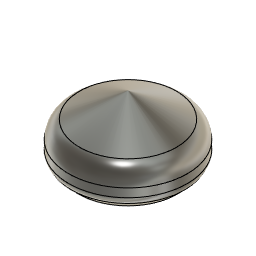
ORS (Autodesk Fusion 360 archive; units mm, degrees)
design "ORS_Button_Pin"
Autodesk Fusion 360 part; units mm, degrees
sketch "Main Body Sketch" plane through (0, 0, 0) normal (0, 0, 1) x (1, 0, 0)
  circle A0 centre (0, 0) radius 3
  dimension "d1" = 6
  constraint coincident A0.centre origin
  measures "d1" diameter of A0
extrude "Extrude1" add sketch "Main Body Sketch" along normal blind 1.75
sketch "Pin Point Sketch" plane through (0, 0, 0) normal (0, 1, 0) x (1, 0, 0)
  line L0 (-3, -1.75) -> (3, -1.75)
  line L1 (3, -1.75) -> (0, -3.29)
  line L2 (0, -3.29) -> (0, -1.75)
  dimension "d4" = 1.54
  constraint coincident L0.end L1.start
  constraint midpoint L0 L2.end
  constraint perpendicular L0 L2
  measures "d4" distance of L1.end L2.end
revolve "Revolve1" add sketch "Pin Point Sketch" angle 360 about axis through (0, 0, 0) along (0, 0, -1)
fillet "Fillet1" radius 1 1 edges at (-2.797, -1.0848, 1.75)
chamfer "Chamfer1" distance 0.5 angle 45 1 edges at (-2.797, -1.0848, 0)
fillet "Fillet2" radius 0.5 1 edges at (-2.797, 1.0848, 0.5)
named bodies: "ORS_Button_Pin"

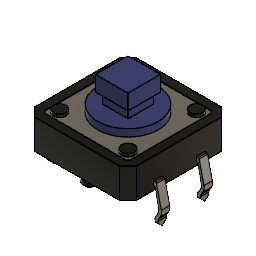
design "OMRON_B3F_5050 v3"
Autodesk Fusion 360 part; units mm, degrees
sketch "Sketch2" plane through (0, 0, 0) normal (0, 0, 1) x (1, 0, 0)
  line L0 (6, 6) -> (-6, 6)
  line L1 (-6, 6) -> (-6, -6)
  line L2 (-6, -6) -> (6, -6)
  line L3 (6, -6) -> (6, 6)
  line L4 (6, 6) -> (-6, -6) construction
  line L5 (-6, 6) -> (6, -6) construction
  circle A0 centre (0.0239, -4.5) radius 0.8
  circle A1 centre (0.0239, 4.5) radius 0.8
  line L6 (-6, 0) -> (6, 0) construction
  line L7 (0, 6) -> (0, -6) construction
  circle A2 centre (0, 0) radius 3.55
  line L8 (1.9, 1.9) -> (-1.9, 1.9)
  line L9 (-1.9, 1.9) -> (-1.9, -1.9)
  line L10 (-1.9, -1.9) -> (1.9, -1.9)
  line L11 (1.9, -1.9) -> (1.9, 1.9)
  line L12 (1.9, 1.9) -> (-1.9, -1.9) construction
  line L13 (-1.9, 1.9) -> (1.9, -1.9) construction
  line L14 (5, 6) -> (6, 5)
  line L15 (-6, 5) -> (-5, 6)
  line L16 (-6, -5) -> (-5, -6)
  line L17 (6, -5) -> (5, -6)
  line L18 (-5, 5) -> (5, 5)
  line L19 (5, 5) -> (5, -5)
  line L20 (5, -5) -> (-5, -5)
  line L21 (-5, -5) -> (-5, 5)
  line L22 (-5, 5) -> (5, -5) construction
  line L23 (5, 5) -> (-5, -5) construction
  line L24 (-4, 4) -> (4, 4) construction
  line L25 (4, 4) -> (4, -4) construction
  line L26 (4, -4) -> (-4, -4) construction
  line L27 (-4, -4) -> (-4, 4) construction
  line L28 (-4, 4) -> (4, -4) construction
  line L29 (4, 4) -> (-4, -4) construction
  circle A3 centre (-4, 4) radius 0.75
  circle A4 centre (4, 4) radius 0.75
  circle A5 centre (4, -4) radius 0.75
  circle A6 centre (-4, -4) radius 0.75
  line L30 (-4.75, -5) -> (-5, -4.75)
  line L31 (-4.75, 5) -> (-5, 4.75)
  line L32 (4.75, 5) -> (5, 4.75)
  line L33 (5, -4.75) -> (4.75, -5)
  line L34 (-6, -2.5) -> (6, -2.5) construction
  line L35 (-6, 2.5) -> (6, 2.5) construction
  line L36 (-1.5, -1.5) -> (1.5, -1.5)
  line L37 (1.5, -1.5) -> (1.5, 1.5)
  line L38 (1.5, 1.5) -> (-1.5, 1.5)
  line L39 (-1.5, 1.5) -> (-1.5, -1.5)
  line L40 (-1.5, -1.5) -> (1.5, 1.5) construction
  line L41 (1.5, -1.5) -> (-1.5, 1.5) construction
  dimension "d3" = 12
  dimension "d4" = 12
  dimension "d5" = 9
  dimension "d6" = 1.6
  dimension "d7" = 7.1
  dimension "d12" = 3.8
  dimension "d13" = 3.8
  dimension "d16" = 1
  dimension "d17" = 1
  dimension "d18" = 1
  dimension "d19" = 1
  dimension "d20" = 10
  dimension "d21" = 10
  dimension "d22" = 8
  dimension "d23" = 8
  dimension "d24" = 1.5
  dimension "d30" = 0.25
  dimension "d31" = 0.25
  dimension "d32" = 0.25
  dimension "d33" = 0.25
  dimension "d37" = 5
  dimension "d46" = 3
  dimension "d47" = 3
  constraint perpendicular L0 L1
  constraint parallel L0 L2
  constraint parallel L1 L3
  constraint horizontal L0
  constraint coincident L4 A2.centre
  constraint coincident L5 A2.centre
  constraint coincident A2.centre origin
  constraint midpoint L1 L6.start
  constraint midpoint L3 L6.end
  constraint midpoint L0 L7.start
  constraint midpoint L2 L7.end
  constraint equal A0 A1
  constraint symmetric A0 A1 L6
  constraint perpendicular L8 L9
  constraint parallel L8 L10
  constraint parallel L9 L11
  constraint horizontal L8
  constraint coincident L12 A2.centre
  constraint coincident L13 A2.centre
  constraint coincident L0 L14.start
  constraint coincident L3 L14.end
  constraint perpendicular L4 L14
  constraint coincident L1 L15.start
  constraint coincident L0 L15.end
  constraint perpendicular L5 L15
  constraint coincident L1 L16.start
  constraint coincident L2 L16.end
  constraint perpendicular L4 L16
  constraint coincident L3 L17.start
  constraint coincident L2 L17.end
  constraint perpendicular L5 L17
  constraint perpendicular L18 L19
  constraint parallel L18 L20
  constraint parallel L19 L21
  constraint horizontal L18
  constraint coincident L22 A2.centre
  constraint coincident L23 A2.centre
  constraint perpendicular L24 L25
  constraint parallel L24 L26
  constraint parallel L25 L27
  constraint horizontal L24
  constraint coincident L28 A2.centre
  constraint coincident L29 A2.centre
  constraint coincident L24.start L27.end
  constraint coincident L24.end L25.start
  constraint coincident L25.end L26.start
  constraint coincident L26.end L27.start
  constraint equal A4 A5
  constraint equal A3 A4
  constraint equal A3 A6
  constraint coincident L20 L30.start
  constraint coincident L21 L30.end
  constraint perpendicular L4 L30
  constraint coincident L18 L31.start
  constraint coincident L21 L31.end
  constraint perpendicular L5 L31
  constraint coincident L18 L32.start
  constraint coincident L19 L32.end
  constraint perpendicular L23 L32
  constraint coincident L19 L33.start
  constraint coincident L20 L33.end
  constraint perpendicular L22 L33
  constraint coincident L1 L34.start
  constraint coincident L3 L34.end
  constraint perpendicular L3 L34
  constraint coincident L1 L35.start
  constraint coincident L3 L35.end
  constraint perpendicular L3 L35
  constraint symmetric L6 L34 L35
  constraint perpendicular L36 L37
  constraint parallel L36 L38
  constraint parallel L37 L39
  constraint horizontal L36
  constraint coincident L40 A2.centre
  constraint coincident L41 A2.centre
  measures "d3" distance of L1.end L2.end
  measures "d4" distance of L0.end L1.end
  measures "d5" distance of A0.centre A1.centre
  measures "d6" diameter of A0
  measures "d7" diameter of A2
  measures "d12" distance of L9.end L10.end
  measures "d13" distance of L8.end L9.end
  measures "d16" distance of L3 L14.start
  measures "d17" distance of L2 L17.start
  measures "d18" distance of L1 L16.end
  measures "d19" distance of L1 L15.end
  measures "d20" distance of L19.end L20.end
  measures "d21" distance of L18.end L19.end
  measures "d22" distance of L25.end L26.end
  measures "d23" distance of L24.end L25.end
  measures "d24" diameter of A4
  measures "d30" distance of L21 L30.start
  measures "d31" distance of L21 L31.start
  measures "d32" distance of L19 L32.start
  measures "d33" distance of L19 L33.end
  measures "d37" distance of L34 L35
  measures "d46" distance of L37.end L38.end
  measures "d47" distance of L36.end L37.end
extrude "Extrude1" add sketch "Sketch2" along normal blind 3.5 contours L0 L1 L2 L3 L14 L15 L16 L17 | A0 L20 | A0 A1 L18 L19 L20 L21 L30 L31 L32 L33 | A0 L20 | L20 L21 L30 | L19 L20 L33 | L18 L21 L31 | L18 L19 L32 | A1 L18 | A1 L18 | A2 | L8 L9 L10 L11 | A3 | A4 | A5 | A6 | L36 L37 L38 L39
sketch "Sketch3" plane through (0, 0, 0) normal (0, 1, 0) x (1, 0, 0)
  line L0 (0, 0) -> (0.0239, -6.3307) construction
  constraint coincident L0.start origin
ref_plane "WorkPlane1" through (0, 2.5, 0) normal (0, -1, 0) x (1, 0, 0)
extrude "Extrude2" add sketch "Sketch2" along normal blind 4.3 contours A2 | L8 L9 L10 L11 | L36 L37 L38 L39
extrude "Extrude3" add sketch "Sketch2" along normal blind 7.3 contours L36 L37 L38 L39
extrude "Extrude4" cut sketch "Sketch2" against normal blind 0.05 from surface at 3.5 contours A0 L20 | A0 A1 L18 L19 L20 L21 L30 L31 L32 L33 | A1 L18 picked at (0.2424, -4.6252) picked at (0.2531, 4.6214)
extrude "Extrude5" add 4 faces at (3.875, -4.2165, 3.5) (-4.0523, -4.2331, 3.5) (3.946, 3.7673, 3.5) (-4.0268, 4.1955, 3.5) along direction (0, 0, 1) blind 0.3
extrude "Extrude6" add sketch "Sketch2" against normal blind 1.571 contours A0 L20 | A0 L20 | A1 L18 | A1 L18
extrude "Extrude8" add sketch "Sketch2" against normal blind 1.8 from surface at 7.3 contours L8 L9 L10 L11
chamfer "Chamfer1" distance 0.3 angle 45 2 edges at (-0.722, -4.2107, -1.571) (-0.722, 4.7893, -1.571)
sketch "Sketch4" plane through (0, 0, 0) normal (0, 1, 0) x (1, 0, 0)
  line L0 (6, 0) -> (6, -3.5)
  line L1 (6, -0.9872) -> (6.2142, -0.9872)
  arc A0 (6.2142, -0.9872) -> (6.3353, -0.8912) centre (6.2142, -0.8628) ccw
  line L2 (6.3353, -0.8912) -> (6.9041, 1.5338)
  arc A1 (6.9041, 1.5338) -> (6.7972, 2.2307) centre (5.9848, 1.7494) ccw
  line L3 (6.7972, 2.2307) -> (6.5799, 2.5974)
  arc A2 (6.509, 2.856) -> (6.5799, 2.5974) centre (7.0164, 2.856) ccw
  line L4 (6.509, 2.856) -> (6.509, 3.5738)
  line L5 (6.509, 3.5738) -> (6.1441, 3.5738)
  line L6 (6.1441, 3.5738) -> (6.1441, 2.7322)
  arc A3 (6.1441, 2.7322) -> (6.1774, 2.6106) centre (6.3827, 2.7322) ccw
  line L7 (6.1774, 2.6106) -> (6.5404, 1.9981)
  arc A4 (6.5945, 1.6858) -> (6.5404, 1.9981) centre (6.1568, 1.7708) ccw
  line L8 (6.5945, 1.6858) -> (6.1731, -0.4862)
  line L9 (6.1731, -0.4862) -> (6, -0.4862)
  line L10 (6, -0.4862) -> (6, -0.9872)
  constraint coincident L0 L1.start
  constraint perpendicular L0 L1
  constraint tangent L1 A0
  constraint tangent L2 A1
  constraint tangent L3 A2
  constraint vertical L4
  constraint perpendicular L4 L5
  constraint perpendicular L5 L6
  constraint tangent L6 A3
  constraint parallel L3 L7
  constraint tangent L7 A4
  constraint coincident L0 L9.end
  constraint perpendicular L0 L9
  constraint tangent A0 L2
  constraint tangent A4 L8
  constraint tangent A1 L3
  constraint tangent A3 L7
  constraint tangent A2 L4
extrude "Extrude7" add sketch "Sketch4" along normal mid plane 1 from surface at 2.5
mirror "Mirror1" about plane through (0, 0, 0) normal (0, 1, 0) of "Extrude7"
mirror "Mirror2" about plane through (0, 0, 0) normal (1, 0, 0) of "Extrude7", "Mirror1"
chamfer "Chamfer2" distance 0.5 angle 45 8 edges at (6.3266, -3, -3.5738) (-6.3266, 2, -3.5738) (6.3266, 2, -3.5738) (-6.3266, -3, -3.5738) (6.3266, -2, -3.5738) (6.3266, 3, -3.5738) (-6.3266, -2, -3.5738) (-6.3266, 3, -3.5738)
